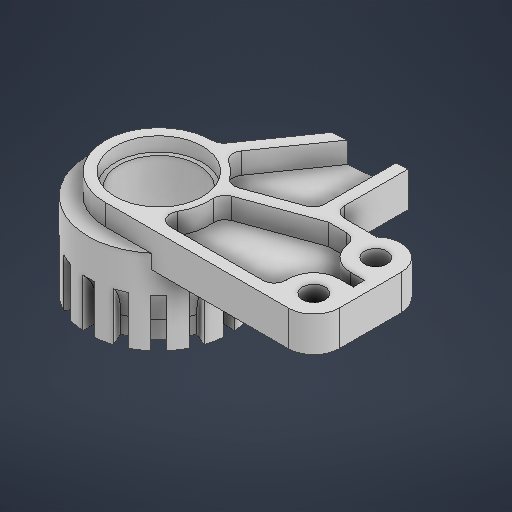
# Autodesk Inventor part: b6
Saved by Autodesk Inventor 2025.4 (Build 294407000, 407)
## iProperties
Created: 2026-05-15
Part Number: b6
Material: Generic
Document SubType Name: Modeling
Designer: VuQuan
Density: 1 g/cm^3
Appearance: Default
Author: VuQuan
Autodesk Inventor part; units mm, degrees
ref_plane "YZ Plane" through (0, 0, 0) normal (1, 0, 0) x (0, 1, 0)
ref_plane "XZ Plane" through (0, 0, 0) normal (0, 1, 0) x (-1, 0, 0)
sketch "Sketch1" plane through (0, 0, 0) normal (0, 1, 0) x (-1, 0, 0)
  circle A0 centre (0, 0) radius 19
  line L0 (0, 19) -> (-65, 19)
  line L1 (-74, 10) -> (-74, -12)
  arc A1 (-74, -12) -> (-58.7751, -18.5) centre (-65, -12) ccw
  line L2 (-58.7751, -18.5) -> (-47.5, -18.5)
  arc A2 (-43.5, -22.5) -> (-47.5, -18.5) centre (-47.5, -22.5) ccw
  line L3 (-43.5, -22.5) -> (-43.5, -45)
  line L4 (-43.5, -45) -> (-18.6145, -42.6104)
  line L5 (-18.6145, -42.6104) -> (-3.2766, -20.7057)
  arc A3 (0, -19) -> (-3.2766, -20.7057) centre (0, -23) ccw
  line L6 (0, 19) -> (0, -19) construction
  arc A4 (-65, 19) -> (-74, 10) centre (-65, 10) ccw
  point P0 (-74, 19)
  dimension "d0" = 38
  dimension "d1" = 74
  dimension "d2" = 35
  dimension "d3" = 25
  dimension "d4" = 43.5
  dimension "d5" = 9
  dimension "d6" = 64
  dimension "d7" = 37.5
  dimension "d8" = 4
  dimension "d9" = 22
  constraints: 14 end point, 11 point on circle, 8 tangent, 5 centre point, 3 point on line, 2 equal radius, 2 vertical, 1 coincident, 1 horizontal, 1 parallel, 1 perpendicular
  measures "d0" diameter of A0
  measures "d1" distance of L0.start point (-74, 19)
  measures "d2" angle of L6 L5
  measures "d3" distance of L3.end L4.end
  measures "d4" distance from line of L3.end L6
  measures "d5" radius of A4
  measures "d6" vertical distance of L3.end point (-74, 19)
  measures "d7" distance from line of point (-74, 19) L2
  measures "d8" radius of A2
  measures "d9" distance of A1.centre A4.centre
extrude "Extrusion1" add sketch "Sketch1" along normal blind 12.5
ref_plane "Work Plane1" through (0, 5, 0) normal (0, 1, 0) x (1, 0, 0)
sketch "Sketch2" plane through (0, 5, 0) normal (0, 1, 0) x (1, 0, 0)
  arc A0 (0, 19) -> (0, -19) centre (0, 0) ccw projected
  circle A1 centre (0, 0) radius 25
  dimension "d13" = 50
  constraints: 1 centre point, 1 coincident
  measures "d13" diameter of A1
extrude "Extrusion2" add sketch "Sketch2" against normal blind 30
sketch "Sketch3" plane through (0, -25, 0) normal (0, -1, 0) x (1, 0, 0)
  circle A0 centre (0, 0) radius 25 projected
  circle A1 centre (0, 0) radius 14
  dimension "d16" = 28
  constraints: 1 centre point, 1 coincident
  measures "d16" diameter of A1
extrude "Extrusion3" cut sketch "Sketch3" against normal through all contours A1
sketch "Sketch4" plane through (0, 12.5, 0) normal (0, 1, 0) x (1, 0, 0)
  arc A0 (0, 19) -> (0, -19) centre (0, 0) ccw projected
  circle A1 centre (0, 0) radius 15.5
  dimension "d19" = 31
  constraints: 1 centre point, 1 coincident
  measures "d19" diameter of A1
extrude "Extrusion4" cut sketch "Sketch4" against normal blind 5
sketch "Sketch5" plane through (0, 0, 0) normal (0, 0, 1) x (1, 0, 0)
  line L0 (-20, -25) -> (-20, -19)
  arc A0 (-20, -19) -> (-25, -7.8197) centre (-35, -19) ccw
  line L1 (-25, -25) -> (25, -25) projected
  line L2 (-25, 5) -> (-25, -25) projected
  point P0 (0, 0)
  point P1 (0, -25)
  dimension "d22" = 15
  dimension "d23" = 6
  dimension "d24" = 20
  constraints: 2 end point, 2 point on circle, 2 point on line, 1 centre point, 1 midpoint, 1 tangent, 1 vertical
  measures "d22" radius of A0
  measures "d23" vertical distance of L0.start A0.centre
  measures "d24" distance of point (0, -25) L0.start
extrude "Extrusion5" cut sketch "Sketch5" along normal mid plane 4
pattern_circular "Circular Pattern1" count 16 over 360 about axis through (0, -10, 0) along (0, 1, 0) of "Extrusion5"
sketch "Sketch6" plane through (0, 12.5, 0) normal (0, 1, 0) x (1, 0, 0)
  circle A0 centre (0, 0) radius 15.5 projected
  line L0 (0, -19) -> (65, -19) projected
  arc A1 (65, -19) -> (74, -10) centre (65, -10) ccw projected
  line L1 (74, -10) -> (74, 12) projected
  arc A2 (74, 12) -> (58.7751, 18.5) centre (65, 12) ccw projected
  line L2 (58.7751, 18.5) -> (47.5, 18.5) projected
  line L3 (43.5, 22.5) -> (43.5, 45) projected
  line L4 (43.5, 45) -> (18.6145, 42.6104) projected
  line L5 (18.6145, 42.6104) -> (3.2766, 20.7057) projected
  line L6 (23.8495, 43.1131) -> (8.3469, 20.973)
  arc A3 (8.3469, 20.973) -> (9.5101, 15.2826) centre (11.6235, 18.6787) ccw
  arc A4 (14.5943, 10.536) -> (9.5101, 15.2826) centre (0, 0) ccw
  arc A5 (14.5943, 10.536) -> (19.2055, 9.1186) centre (17.8374, 12.8774) ccw
  line L7 (19.2055, 9.1186) -> (36.8681, 15.5472)
  line L8 (39.5, 19.306) -> (39.5, 44.6159)
  arc A6 (36.8681, 15.5472) -> (39.5, 19.306) centre (35.5, 19.306) ccw
  line L9 (52.0385, -15) -> (19.0526, -15)
  arc A7 (15.5885, -9) -> (19.0526, -15) centre (19.0526, -11) ccw
  arc A8 (20.5736, 5.3598) -> (17.9523, 1.3099) centre (21.9417, 1.601) ccw
  line L10 (20.5736, 5.3598) -> (45.686, 14.5)
  line L11 (45.686, 14.5) -> (52.0868, 14.5)
  arc A9 (56.0601, 10.9615) -> (52.0868, 14.5) centre (52.0868, 10.5) ccw
  arc A10 (56.0601, 10.9615) -> (65, 3) centre (65, 12) ccw
  arc A11 (65, -1) -> (56.0267, -10.6923) centre (65, -10) ccw
  arc A12 (52.0385, -15) -> (56.0267, -10.6923) centre (52.0385, -11) ccw
  circle A13 centre (65, 12) radius 4
  circle A14 centre (65, -10) radius 4
  arc A15 (15.5885, -9) -> (17.9523, 1.3099) centre (0, 0) ccw
  line L12 (0, 0) -> (34.3054, 12.4861) construction
  line L13 (65, 3) -> (70, 3)
  line L14 (70, 3) -> (70, -1)
  line L15 (70, -1) -> (65, -1)
  line L16 (-45.2307, 0) -> (96.3758, 0) projected
  circle A16 centre (0, 0) radius 14 projected
  dimension "d30" = 4
  dimension "d31" = 4
  dimension "d32" = 4
  dimension "d34" = 8
  dimension "d35" = 4
  dimension "d36" = 4
  dimension "d37" = 4
  dimension "d38" = 20
  dimension "d39" = 4
  dimension "d40" = 4
  constraints: 22 point on circle, 20 end point, 16 tangent, 13 centre point, 10 equal radius, 4 coincident, 4 parallel, 3 horizontal, 2 concentric, 2 point on line, 1 perpendicular, 1 other
  measures "d30" radius of A3
  measures "d31" distance between parallel lines of L5 L6
  measures "d32" distance between parallel lines of L3 L8
  measures "d34" diameter of A13
  measures "d35" distance between parallel lines of L1 L14
  measures "d36" distance between parallel lines of L0 L9
  measures "d37" distance between parallel lines of L10 L7
  measures "d38" angle of L12 L16
  measures "d39" distance between parallel lines of L2 L11
  measures "d40" radial gap between concentric circles of A4 A16
extrude "Extrusion6" cut sketch "Sketch6" against normal through all contours A13 | A14
extrude "Extrusion7" cut sketch "Sketch6" against normal up to surface (7.5 mm away) contours A15 A8 L10 L11 A9 A10 L13 L14 L16 | L16 L14 L15 A11 A12 L9 A7 A15 | L8 A6 L7 A5 A4 A3 L6 L4
body "Solid1"
